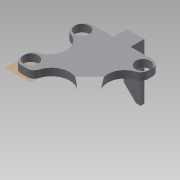
# Autodesk Inventor part: 20_Schlitten
Saved by Autodesk Inventor 2015 (Build 190159000, 159)
## iProperties
Created: 2016-03-06
Part Number: 20_Schlitten
Material: Generisch
Document SubType Name: Modeling
Designer: Bene
Density: 1 g/cm^3
Appearance: Vorgabe
Author: Bene
Autodesk Inventor part; units mm, degrees
ref_plane "YZ Plane" through (0, 0, 0) normal (1, 0, 0) x (0, 1, 0)
ref_plane "XZ Plane" through (0, 0, 0) normal (0, 1, 0) x (-1, 0, 0)
ref_plane "Arbeitsebene1" through (0, 0, -6) normal (0, 0, 1) x (1, 0, 0)
sketch "Skizze1" plane through (0, 0, -6) normal (0, 0, 1) x (1, 0, 0)
  circle A0 centre (0, 42) radius 6 projected
  circle A1 centre (50, 42) radius 6 projected
  circle A2 centre (50, 0) radius 6 projected
  circle A3 centre (0, 0) radius 6 projected
  line L0 (6.489, 48.9995) -> (6.489, 49.9028) projected
  line L1 (6.489, 49.9028) -> (-6, 49.9028) projected
  line L2 (-6, 49.9028) -> (-6, -8.0972) projected
  line L3 (-6, -8.0972) -> (5.7305, -8.0972) projected
  line L4 (5.7305, -8.0972) -> (5.7305, -4.6433) projected
  line L5 (5.7305, -4.6433) -> (25.1643, -4.6433) projected
  line L6 (25.1643, -4.6433) -> (13.6183, -0.9927) projected
  line L7 (13.6183, -0.9927) -> (6.9629, 3.2) projected
  line L8 (6.9629, 3.2) -> (-0.5, 23.5649) projected
  line L9 (-0.5, 23.5649) -> (2.346, 34.9379) projected
  line L10 (2.346, 34.9379) -> (18.55, 40.876) projected
  line L11 (18.55, 40.876) -> (19.7446, 48.9995)
  line L12 (19.7446, 48.9995) -> (6.489, 48.9995) projected
  circle A4 centre (0, 42) radius 3.2 projected
  circle A5 centre (0, 0) radius 3.2 projected
  line L13 (-6, -8.0972) -> (56, -8.0972)
  line L14 (56, -8.0972) -> (56, 49.9028)
  line L15 (56, 49.9028) -> (-6, 49.9028)
  line L16 (-6, 49.9028) -> (-6, -8.0972)
  circle A6 centre (25, 19) radius 21 projected
  line L17 (22.1022, 54.5009) -> (31.9971, 38.8) construction
  line L18 (31.9971, 54.5009) -> (22.1022, 38.8) construction
  point P0 (0, 0)
  constraints: 14 end point, 2 parallel, 1 horizontal, 1 perpendicular
extrude "Extrusion1" add sketch "Skizze1" along normal blind 6 contours L2 L1 L0 L12 L11 L10 L9 L8 L7 L6 L5 L4 L3 | L15 L14 L13 L4 L5 L6 L7 L8 L9 L10 L11 L12 L0 | A6
sketch "Skizze2" plane through (0, 0, 0) normal (0, 0, 1) x (1, 0, 0)
  circle A0 centre (0, 42) radius 6 projected
  circle A1 centre (0, 0) radius 6 projected
  line L0 (56, -8.0972) -> (56, 0) projected
  circle A2 centre (50, 0) radius 6 projected
  line L1 (56, 0) -> (56, 42) projected
  circle A3 centre (50, 42) radius 6 projected
  line L2 (56, 42) -> (56, 49.9028) projected
  line L3 (56, 49.9028) -> (-6, 49.9028) projected
  line L4 (-6, 42) -> (-6, 0) projected
  circle A4 centre (-6, 21) radius 14
  line L5 (56, 0) -> (56, 42) projected
  circle A5 centre (56, 21) radius 14
  line L6 (-6, -8.0972) -> (56, -8.0972) projected
  circle A6 centre (25, -8.0972) radius 15
  line L7 (-6, -8.0972) -> (56, -8.0972) projected
  line L8 (-6, 49.9028) -> (-6, 42) projected
  line L9 (-6, 42) -> (-6, 0) projected
  line L10 (-6, 0) -> (-6, -8.0972) projected
  point P0 (0, 0)
  dimension "d3" = 28
  dimension "d4" = 28
  dimension "d5" = 30
  constraints: 4 horizontal alignment, 3 centre point, 3 midpoint
  measures "d3" diameter of A4
  measures "d4" diameter of A5
  measures "d5" diameter of A6
extrude "Extrusion2" cut sketch "Skizze2" against normal blind 6 contours A4 L4 | L4 A4 | A5 L1 | L1 A5 | A6 L6 | L6 A6
fillet "Rundung1" radius 6 10 edges at (56, 35, -3) (56, 7, -3) (56, 49.9028, -3) (56, -8.0972, -3) (40, -8.0972, -3) (10, -8.0972, -3) (-6, -8.0972, -3) (-6, 7, -3) (-6, 35, -3) (-6, 49.9028, -3)
sketch "Skizze4" plane through (0, 0, 0) normal (0, 0, 1) x (1, 0, 0)
  arc A0 (0, 49.9028) -> (-6, 43.9028) centre (0, 43.9028) ccw projected
  line L0 (-6, 43.9028) -> (-6, 42) projected
  circle A1 centre (0, 42) radius 6 projected
  line L1 (-6, 42) -> (-6, 40.0788) projected
  arc A2 (-6, 40.0788) -> (-1.8, 34.3551) centre (0, 40.0788) ccw projected
  arc A3 (-1.8, 7.6449) -> (-1.8, 34.3551) centre (-6, 21) ccw projected
  arc A4 (-1.8, 7.6449) -> (-6, 1.9212) centre (0, 1.9212) ccw projected
  line L2 (-6, 1.9212) -> (-6, 0) projected
  circle A5 centre (0, 0) radius 6 projected
  line L3 (-6, 0) -> (-6, -2.0972) projected
  arc A6 (-6, -2.0972) -> (0, -8.0972) centre (0, -2.0972) ccw projected
  line L4 (0, -8.0972) -> (4.8754, -8.0972) projected
  arc A7 (4.8754, -8.0972) -> (10.6253, -3.8115) centre (4.8754, -2.0972) ccw projected
  arc A8 (39.3747, -3.8115) -> (10.6253, -3.8115) centre (25, -8.0972) ccw projected
  arc A9 (39.3747, -3.8115) -> (45.1246, -8.0972) centre (45.1246, -2.0972) ccw projected
  line L5 (45.1246, -8.0972) -> (50, -8.0972) projected
  arc A10 (50, -8.0972) -> (56, -2.0972) centre (50, -2.0972) ccw projected
  line L6 (56, -2.0972) -> (56, 0) projected
  circle A11 centre (50, 0) radius 6 projected
  line L7 (56, 0) -> (56, 1.9212) projected
  arc A12 (56, 1.9212) -> (51.8, 7.6449) centre (50, 1.9212) ccw projected
  arc A13 (51.8, 34.3551) -> (51.8, 7.6449) centre (56, 21) ccw projected
  arc A14 (51.8, 34.3551) -> (56, 40.0788) centre (50, 40.0788) ccw projected
  line L8 (56, 40.0788) -> (56, 42) projected
  circle A15 centre (50, 42) radius 6 projected
  line L9 (56, 42) -> (56, 43.9028) projected
  arc A16 (56, 43.9028) -> (50, 49.9028) centre (50, 43.9028) ccw projected
  line L10 (50, 49.9028) -> (0, 49.9028) projected
  line L11 (6.6, 89.7038) -> (6.6, 65.7038) projected
  line L12 (6.6, 65.7038) -> (31.6, 65.7038) projected
  line L13 (31.6, 65.7038) -> (31.6, 89.7038) projected
  line L14 (31.6, 89.7038) -> (6.6, 89.7038) projected
  circle A17 centre (29.6, 87.7038) radius 1.05 projected
  circle A18 centre (29.6, 75.2038) radius 1.05 projected
  circle A19 centre (8.6, 75.2038) radius 1.05 projected
  circle A20 centre (8.6, 87.7038) radius 1.05 projected
  line L15 (27.8, 85.1038) -> (26.58, 85.1038) projected
  line L16 (27.8, 84.3038) -> (27.8, 85.1038) projected
  line L17 (26.58, 84.3038) -> (27.8, 84.3038) projected
  line L18 (26.58, 85.1038) -> (26.58, 84.3038) projected
  line L19 (50, 49.9028) -> (0, 49.9028) projected
  line L20 (31.6, 49.9028) -> (6.6, 49.9028)
  line L21 (6.6, 49.9028) -> (6.6, 51.9028)
  line L22 (6.6, 51.9028) -> (31.6, 51.9028)
  line L23 (31.6, 51.9028) -> (31.6, 49.9028)
  point P0 (0, 0)
  dimension "d13" = 2
  constraints: 8 end point, 4 horizontal alignment, 2 parallel, 1 horizontal, 1 perpendicular, 1 point on line
  measures "d13" distance of L20.end L21.end
extrude "Extrusion4" add sketch "Skizze4" against normal blind 6 contours L21 L22 L23 L10
